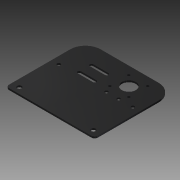
# Autodesk Inventor part: motor_mount_v2
Saved by Autodesk Inventor 2014 (Build 180170000, 170)
## iProperties
Created: 2013-07-17
Part Number: motor_mount_v2
Material: Steel, Mild
Document SubType Name: Modeling
Designer: Edward
Density: 7.86 g/cm^3
Appearance: Lacquer - Black
d0: 145.000 mm
d1: 130.000 mm
d2: 65.000 mm
d3: 72.500 mm
d4: 2.657 mm
d5: 0.00 deg
d6: 25.000 mm
d7: 5.500 mm
d8: 30.000 mm
d9: 40.000 mm
d11: 0.00 deg
d12: 2.000 ul
d14: 20.000 mm
d15: 7.140 mm
d16: 5.500 mm
d17: 64.600 mm
d18: 10.000 mm
d19: 12.000 mm
d21: 12.000 mm
d23: 0.00 deg
d24: 2.000 ul
d26: 121.000 mm
d27: 23.000 mm
d28: 29.000 mm
d29: 4.000 mm
d30: 15.500 mm
d31: 15.500 mm
d36: 45.000 mm
d38: 0.00 deg
d39: 25.000 mm
d41: 5.500 mm
d42: 74.500 mm
d43: 90.000 mm
d45: 0.00 deg
d49: 2.000 ul
d51: 31.000 mm
d52: 2.000 ul
d54: 31.000 mm
Author: Edward
Autodesk Inventor part; units mm, degrees
ref_plane "YZ Plane" through (0, 0, 0) normal (1, 0, 0) x (0, 1, 0)
ref_plane "XZ Plane" through (0, 0, 0) normal (0, 1, 0) x (-1, 0, 0)
ref_plane "XY Plane" through (0, 0, 0) normal (0, 0, 1) x (1, 0, 0)
sketch "Sketch1" plane through (0, 0, 0) normal (0, 0, 1) x (1, 0, 0)
  line L0 (-72.5, 65) -> (72.5, 65)
  line L1 (72.5, 65) -> (72.5, -65)
  line L2 (72.5, -65) -> (-72.5, -65)
  line L3 (-72.5, -65) -> (-72.5, 65)
  point P0 (0, 0)
  dimension "d0" = 145
  dimension "d1" = 130
  dimension "d2" = 65
  dimension "d3" = 72.5
  constraints: 8 end point, 2 parallel, 1 horizontal, 1 perpendicular
  measures "d0" distance of L1.end L2.end
  measures "d1" distance of L0.end L1.end
  measures "d2" distance from line of L0 point (0, 0)
  measures "d3" distance from line of L3 point (0, 0)
extrude "profile" add sketch "Sketch1" along normal blind 2.6568
sketch "Sketch2" plane through (0, 0, 2.6568) normal (0, 0, 1) x (1, 0, 0)
  line L0 (72.5, 65) -> (-72.5, 65) projected
  line L1 (-72.5, 65) -> (-72.5, -65) projected
  line L2 (-32.5, 35) -> (-7.5, 35) construction
  line L3 (-32.5, 32.25) -> (-7.5, 32.25)
  line L4 (-7.5, 37.75) -> (-32.5, 37.75)
  arc A0 (-32.5, 37.75) -> (-32.5, 32.25) centre (-32.5, 35) ccw
  arc A1 (-7.5, 32.25) -> (-7.5, 37.75) centre (-7.5, 35) ccw
  point P0 (0, 0)
  point P1 (-20, 35)
  dimension "d6" = 25
  dimension "d7" = 5.5
  dimension "d8" = 30
  dimension "d9" = 40
  constraints: 8 end point, 4 point on circle, 4 tangent, 2 centre point, 2 parallel, 1 midpoint
  measures "d6" distance of L2.start L2.end
  measures "d7" diameter of A1
  measures "d8" distance from line of L0 L2.start
  measures "d9" distance from line of L1 L2.start
extrude "x_slots" cut sketch "Sketch2" against normal through all
pattern_linear "Rectangular Pattern1" count 2 spacing 20 along (0, -1, 0) of "x_slots"
sketch "Sketch3" plane through (0, 0, 2.6568) normal (0, 0, 1) x (1, 0, 0)
  line L0 (-72.5, 65) -> (-72.5, -65) projected
  line L1 (-72.5, -65) -> (72.5, -65) projected
  circle A0 centre (-60.5, -55) radius 3.57
  circle A1 centre (-60.5, 9.6) radius 2.75
  circle A2 centre (-60.5, 9.6) radius 11.75 construction
  point P0 (0, 0)
  dimension "d15" = 7.14
  dimension "d16" = 5.5
  dimension "d17" = 64.6
  dimension "d18" = 10
  dimension "d19" = 12
  dimension "d21" = 12
  constraints: 3 centre point, 1 coincident
  measures "d15" diameter of A0
  measures "d16" diameter of A1
  measures "d17" distance of A0.centre A1.centre
  measures "d18" distance from line of L1 A0.centre
  measures "d19" distance from line of L0 A0.centre
  measures "d21" distance from line of L0 A2.centre
extrude "Extrusion3" cut sketch "Sketch3" against normal through all
pattern_linear "Rectangular Pattern2" count 2 spacing 121 along (1, 0, 0) of "Extrusion3"
sketch "Sketch4" plane through (0, 0, 2.6568) normal (0, 0, 1) x (1, 0, 0)
  line L0 (72.5, 65) -> (-72.5, 65) projected
  line L1 (72.5, -65) -> (72.5, 65) projected
  circle A0 centre (27.5, 36) radius 11.5
  circle A1 centre (12, 51.5) radius 2
  circle A2 centre (43, 51.5) radius 2
  circle A3 centre (12, 20.5) radius 2
  circle A4 centre (43, 20.5) radius 2
  point P0 (0, 0)
  dimension "d27" = 23
  dimension "d28" = 29
  dimension "d29" = 4
  dimension "d30" = 15.5
  dimension "d31" = 15.5
  dimension "d36" = 45
  dimension "d51" = 31
  dimension "d54" = 31
  constraints: 5 centre point, 1 horizontal, 1 vertical, 6 other
  measures "d27" diameter of A0
  measures "d28" distance from line of L0 A0.centre
  measures "d29" diameter of A1
  measures "d30" horizontal distance of A0.centre A1.centre
  measures "d31" horizontal distance of A1.centre A0.centre
  measures "d36" distance from line of L1 A0.centre
  measures "d51" distance of A1.centre A2.centre
  measures "d54" distance of A1.centre A3.centre
extrude "nema17_mount" cut sketch "Sketch4" against normal through all
fillet "Fillet1" radius 25 2 edges at (72.5, 65, 1.3284) (-72.5, 65, 1.3284)
sketch "Sketch5" plane through (0, 0, 2.6568) normal (0, 0, 1) x (1, 0, 0)
  line L0 (-72.5, 65) -> (-72.5, -65) projected
  line L1 (-72.5, -65) -> (72.5, -65) projected
  circle A0 centre (17.5, 9.5) radius 2.75
  line L2 (47.5, 65) -> (-72.5, 65) projected
  circle A1 centre (37.5, 9.5) radius 2.75
  point P0 (67.5, -65)
  point P1 (-72.5, 60)
  point P2 (-72.5, -60)
  point P3 (-67.5, -65)
  point P4 (0, 0)
  dimension "d41" = 5.5
  dimension "d42" = 74.5
  dimension "d43" = 90
  dimension "d59" = 20
  constraints: 2 centre point, 1 horizontal, 2 other
  measures "d41" diameter of A0
  measures "d42" distance from line of L1 A0.centre
  measures "d43" distance from line of L0 A0.centre
  measures "d59" distance of A0.centre A1.centre
extrude "idler_holes" cut sketch "Sketch5" against normal through all
fillet "Fillet3" radius 5 2 edges at (-72.5, -65, 1.3284) (72.5, -65, 1.3284)
equation "\"d2\" = 0.5 * d1"
equation "\"d3\" = 0.5 * d0"
body "Solid1"
